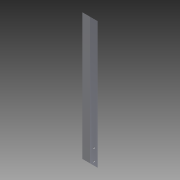
# Autodesk Inventor part: Square Tube 3
Saved by Autodesk Inventor 2013 (Build 170138000, 138)
## iProperties
Created: 2013-01-24
Part Number: Square Tube 3
Material: Aluminum 6061
Document SubType Name: Modeling
Designer: actoennies
Mass: 119.696 g
Surface Area: 560.101 cm^2
Volume: 44.1683 cm^3
Density: 2.71 g/cm^3
Author: actoennies
Autodesk Inventor part; units mm, degrees
ref_plane "YZ Plane" through (0, 0, 0) normal (1, 0, 0) x (0, 1, 0)
ref_plane "XZ Plane" through (0, 0, 0) normal (0, 1, 0) x (-1, 0, 0)
ref_plane "XY Plane" through (0, 0, 0) normal (0, 0, 1) x (1, 0, 0)
sketch "Sketch1" plane through (0, 0, 0) normal (0, 1, 0) x (-1, 0, 0)
  line L0 (0, 0) -> (25.4, 0)
  line L1 (25.4, 0) -> (25.4, 25.4)
  line L2 (25.4, 25.4) -> (0, 25.4)
  line L3 (0, 25.4) -> (0, 0)
  line L4 (1.5875, 23.8125) -> (23.8125, 23.8125)
  line L5 (23.8125, 23.8125) -> (23.8125, 1.5875)
  line L6 (23.8125, 1.5875) -> (1.5875, 1.5875)
  line L7 (1.5875, 1.5875) -> (1.5875, 23.8125)
  dimension "d0" = 25.4
  dimension "d2" = 25.4
  dimension "d3" = 1.5875
  constraints: 16 end point, 4 parallel, 2 perpendicular, 1 horizontal, 3 other
  measures "d0" distance of L1.end L2.end
  measures "d2" distance of L0.end L1.end
  measures "d3" distance between parallel lines of L2 L4
extrude "Extrusion1" add sketch "Sketch1" along normal blind 444.5
sketch "Sketch2" plane through (-25.4, 0, 0) normal (-1, 0, 0) x (0, 0, 1)
  line L0 (0, 444.5) -> (25.4, 444.5) projected
  line L1 (0, 0) -> (0, 444.5) projected
  line L2 (25.4, 444.5) -> (0, 419.1)
  dimension "d6" = 25.4
  constraints: 2 end point, 1 point on line
  measures "d6" distance of L2.end L0.start
extrude "Extrusion2" cut sketch "Sketch2" against normal blind 25.4
sketch "Sketch3" plane through (-25.4, 0, 0) normal (-1, 0, 0) x (0, 0, 1)
  line L0 (25.4, 444.5) -> (0, 419.1) projected
  line L1 (0, 0) -> (25.4, 0) projected
  line L2 (25.4, 0) -> (25.4, 444.5) projected
  line L3 (0, 0) -> (25.4, 25.4)
  constraints: 2 end point, 1 parallel, 1 point on line
extrude "Extrusion3" cut sketch "Sketch3" against normal blind 25.4
sketch "Sketch4" plane through (-25.4, 25.4, 25.4) normal (-1, 0, 0) x (0, 0, 1)
  circle A0 centre (-12.7, 38.1) radius 3.3782 projected
  circle A1 centre (-12.7, 0) radius 3.3782 projected
extrude "Extrusion4" cut sketch "Sketch4" against normal blind 25.4
body "Solid1"
